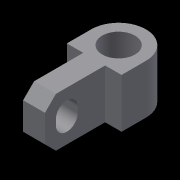
# Autodesk Inventor part: ForearmCuffConnector
Saved by Autodesk Inventor 2015 (Build 190159000, 159)
## iProperties
RuleStatus: InUse
Created: 2014-10-05
Part Number: ForearmCuffConnector
Material: Generic
Document SubType Name: Modeling
Designer: Val
Density: 1 g/cm^3
Appearance: Default
Mass: 0.814558 g
Surface Area: 8.86444 cm^2
Volume: 0.814558 cm^3
BeforeDocSave0: UpdateBoundingBox
CX: 10.00 mm
CY: 20.47 mm
CZ: 9.00 mm
Author: Val
Autodesk Inventor part; units mm, degrees
ref_plane "YZ Plane" through (0, 0, 0) normal (1, 0, 0) x (0, 1, 0)
ref_plane "XZ Plane" through (0, 0, 0) normal (0, 1, 0) x (-1, 0, 0)
ref_plane "XY Plane" through (0, 0, 0) normal (0, 0, 1) x (1, 0, 0)
sketch "TopProfile" plane through (0, 0, 0) normal (0, 0, 1) x (1, 0, 0)
  circle A0 centre (0, 0) radius 3
  circle A1 centre (0, 0) radius 5 construction
  line L0 (-2, -4.4651) -> (-2, -15.4651)
  line L1 (-2, -15.4651) -> (2, -15.4651)
  line L2 (2, -15.4651) -> (2, -4.4651)
  line L3 (-2, -4.4651) -> (2, -4.4651)
  line L4 (2.25, -4.4651) -> (-2.25, -4.4651) construction
  line L5 (5, -4.4651) -> (-5, -4.4651)
  line L6 (5, 0) -> (5, -4.4651)
  line L7 (-5, 0) -> (-5, -4.4651)
  arc A2 (5, 0) -> (-5, 0) centre (0, 0) ccw
  dimension "d0" = 6
  dimension "d1" = 10
  dimension "d3" = 4
  dimension "d5" = 11
  dimension "d8" = 4.5
  dimension "d9" = 0.25
  constraints: 16 end point, 6 point on circle, 3 centre point, 3 tangent, 2 coincident, 2 horizontal, 2 parallel, 2 perpendicular, 2 vertical, 1 collinear, 1 point on line
  measures "d0" diameter of A0
  measures "d1" diameter of A1
  measures "d3" distance of L0.end L1.end
  measures "d5" distance of L0.start L0.end
  measures "d8" distance of L4.start L4.end
  measures "d9" distance of L4.end L0.start
extrude "TopProfileFeature" add sketch "TopProfile" along normal blind 9
chamfer "BodyChamferFeatures" distance 2 angle 45 2 edges at (0, -15.4651, 9) (0, -15.4651, 0)
sketch "MountRail" plane through (2, -13.4651, 9) normal (1, 0, 0) x (0, 0, -1)
  line L0 (0, 0) -> (0, 9) construction
  line L1 (0, 2) -> (9, 2) construction
  arc A0 (5, 0) -> (5, 4) centre (5, 2) ccw
  arc A1 (4, 4) -> (4, 0) centre (4, 2) ccw
  line L2 (5, 4) -> (4, 4)
  line L3 (5, 0) -> (4, 0)
  line L4 (7, -2) -> (2, -2) construction
  line L5 (9, 9) -> (9, 0) construction
  point P0 (9, -2)
  dimension "d41" = 2
  dimension "d43" = 4
  dimension "d44" = 4
  dimension "d55" = 4
  constraints: 6 end point, 4 point on circle, 4 point on line, 4 tangent, 2 centre point, 1 equal radius, 1 horizontal
  measures "d41" radius of A0
  measures "d43" distance from line of L0 A1.centre
  measures "d44" distance between parallel lines of L1 L4
  measures "d55" distance from line of L5 A0.centre
extrude "MountRailFeature" cut sketch "MountRail" against normal through all
